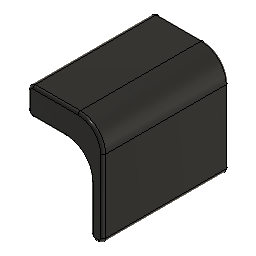
Arm Strap Support1 (Autodesk Fusion 360 design; units mm, degrees)
Autodesk Fusion 360 part; units mm, degrees
sketch "Sketch1" plane through (0, 57.15, 0) normal (0, 1, 0) x (-1, 0, 0)
  line L0 (-4.0409, -6.0198) -> (-4.0409, -7.62)
  line L1 (-4.0409, -7.62) -> (2.9359, -7.62)
  line L2 (2.9359, -7.62) -> (2.9359, -6.0198)
  line L3 (2.9359, -6.0198) -> (-4.0409, -6.0198)
  line L4 (-19.0526, 3.8099) -> (-19.0526, -5.08)
  line L5 (-21.5926, -7.62) -> (-38.1026, -7.62)
  line L6 (-50.8026, -7.62) -> (-50.8026, 6.3499)
  line L7 (-50.8026, 6.3499) -> (-21.5926, 6.3499)
  line L8 (-50.8026, -20.32) -> (-50.8026, -43.18)
  line L9 (-53.3426, -45.72) -> (-54.6126, -45.72)
  line L10 (-57.1526, -43.18) -> (-57.1526, -6.3501)
  line L11 (-44.4526, 6.3499) -> (-50.8026, 6.3499)
  arc A0 (-19.0526, 3.8099) -> (-21.5926, 6.3499) centre (-21.5926, 3.8099) ccw
  arc A1 (-21.5926, -7.62) -> (-19.0526, -5.08) centre (-21.5926, -5.08) ccw
  arc A2 (-53.3426, -45.72) -> (-50.8026, -43.18) centre (-53.3426, -43.18) ccw
  arc A3 (-57.1526, -43.18) -> (-54.6126, -45.72) centre (-54.6126, -43.18) ccw
  arc A4 (-38.1026, -7.62) -> (-50.8026, -20.32) centre (-38.1026, -20.32) ccw
  arc A5 (-44.4526, 6.3499) -> (-57.1526, -6.3501) centre (-44.4526, -6.3501) ccw
  point P0 (-19.0526, -7.62)
  point P1 (-50.8026, -45.72)
  point P2 (-57.1526, -45.72)
  dimension "d1" = 31.75
  dimension "d2" = 38.1
  dimension "d3" = 6.35
  dimension "d4" = 2.54
  dimension "d5" = 2.54
  dimension "d6" = 12.7
  constraint perpendicular L1 L4
  constraint perpendicular L4 L5
  constraint perpendicular L5 L6
  constraint perpendicular L4 L7
  constraint perpendicular L5 L8
  constraint perpendicular L8 L9
  constraint perpendicular L9 L10
  constraint perpendicular L6 L11
  constraint tangent L4 A0
  constraint tangent L7 A0
  constraint coincident P0 L4
  constraint coincident P0 L5
  constraint tangent L4 A1
  constraint tangent L5 A1
  constraint equal A0 A1
  constraint coincident P1 L8
  constraint coincident P1 L9
  constraint tangent L8 A2
  constraint tangent L9 A2
  constraint coincident P2 L9
  constraint coincident P2 L10
  constraint tangent L9 A3
  constraint tangent L10 A3
  constraint equal A2 A3
  constraint coincident L6.start L5
  constraint coincident L6.start L8
  constraint tangent L5 A4
  constraint tangent L8 A4
  constraint tangent L10 A5
  constraint tangent L11 A5
  constraint equal A4 A5
  measures "d1" distance of P0 L6.start
  measures "d2" distance of L6.start P1
  measures "d3" distance of P1 P2
  measures "d4" radius of A0
  measures "d5" radius of A2
  measures "d6" radius of A4
extrude "Extrude1" add sketch "Sketch1" against normal blind 63.5 contours L4 L5 L7 L8 L9 L10 A0 A1 A2 A3 A4 A5
hole "Hole1" at (19.0526, 0, 0) direction (1, 0, 0) diameter 3.429 depth 12.7 tip angle 180
thread "Thread1" "ANSI Unified Screw Threads 0.164(#8) 8-32 UNC 8-32 UNC 2B" major diameter 4.1656 minor diameter 3.4163 pitch 0.7937 angle 60 modelled right hand crest width 0.2341 on face at (23.2859, 0.1707, 1.706) crest through (19.251, -1.7082, 0)
hole "Hole2" at (19.0526, 25.4, 0) direction (1, 0, 0) diameter 3.429 depth 12.7 tip angle 180
thread "Thread2" "ANSI Unified Screw Threads 0.164(#8) 8-32 UNC 8-32 UNC 2B" major diameter 4.1656 minor diameter 3.4163 pitch 0.7937 angle 60 modelled right hand crest width 0.2341 on face at (23.2859, 25.5707, 1.706) crest through (19.251, 23.6918, 0)
hole "Hole3" at (19.0526, 50.8, 0) direction (1, 0, 0) diameter 3.429 depth 12.7 tip angle 180
thread "Thread3" "ANSI Unified Screw Threads 0.164(#8) 8-32 UNC 8-32 UNC 2B" major diameter 4.1656 minor diameter 3.4163 pitch 0.7937 angle 60 modelled right hand crest width 0.2341 on face at (23.2859, 50.9707, 1.706) crest through (19.251, 49.0918, 0)
fillet "Fillet1" radius 1.27 12 edges at (19.0526, -6.35, -0.6351) (19.7966, -6.35, -6.8761) (29.8476, -6.35, -7.62) (47.0829, -6.35, -11.3397) (50.8026, -6.35, -31.75) (51.5466, -6.35, -44.9761) (53.9776, -6.35, -45.72) (56.4087, -6.35, -44.9761) (57.1526, -6.35, -24.7651) (53.4329, -6.35, 2.6301) (33.0226, -6.35, 6.3499) (19.7966, -6.35, 5.6059) 1 faces at (34.7159, 57.15, 1.6932)
sketch "Sketch2" plane through (19.0526, 0, 0) normal (-1, 0, 0) x (0, -1, 0)
  line L0 (-55.88, 3.8099) -> (-55.88, -5.08)
  line L1 (-55.88, -5.08) -> (5.08, -5.08)
  line L2 (5.08, -5.08) -> (5.08, 3.8099)
  line L3 (5.08, 3.8099) -> (-55.88, 3.8099)
  spline S0 degree 3 poles (-1.0037, -1.825) (-1.2209, -1.674) (-1.4071, -1.4829) (-1.6881, -1.048) (-1.7836, -0.8108) (-1.8744, -0.3235) (-1.8728, -0.0789) (-1.7889, 0.3235) (-1.7315, 0.4832) (-1.5758, 0.7763) (-1.4795, 0.909) (-1.3657, 1.0259) knots 0 0 0 0 0.079347 0.079347 0.155456 0.155456 0.228326 0.228326 0.279114 0.279114 0.328226 0.328226 0.328226 0.328226
  arc A0 (1.3657, 1.0259) -> (-1.3657, 1.0259) centre (0, 0) ccw
  spline S1 degree 3 poles (1.3657, 1.0259) (1.5233, 0.864) (1.6469, 0.6723) (1.8197, 0.2427) (1.8634, 0.0074) (1.8602, -0.4776) (1.8092, -0.7228) (1.6412, -1.1248) (1.5443, -1.2864) (1.3049, -1.5826) (1.1624, -1.7147) (1.0037, -1.825) knots 0 0 0 0 0.06777 0.06777 0.138771 0.138771 0.213001 0.213001 0.26909 0.26909 0.326867 0.326867 0.326867 0.326867
  arc A1 (-1.0037, -1.825) -> (1.0037, -1.825) centre (0, 0) ccw
  spline S2 degree 3 poles (-26.4037, -1.825) (-26.6209, -1.674) (-26.8071, -1.4829) (-27.0881, -1.048) (-27.1836, -0.8108) (-27.2744, -0.3235) (-27.2728, -0.0789) (-27.1889, 0.3235) (-27.1315, 0.4832) (-26.9758, 0.7763) (-26.8795, 0.909) (-26.7657, 1.0259) knots 0 0 0 0 0.079347 0.079347 0.155456 0.155456 0.228326 0.228326 0.279114 0.279114 0.328226 0.328226 0.328226 0.328226
  arc A2 (-24.0343, 1.0259) -> (-26.7657, 1.0259) centre (-25.4, 0) ccw
  spline S3 degree 3 poles (-24.0343, 1.0259) (-23.8767, 0.864) (-23.7531, 0.6723) (-23.5803, 0.2427) (-23.5366, 0.0074) (-23.5398, -0.4776) (-23.5908, -0.7228) (-23.7588, -1.1248) (-23.8557, -1.2864) (-24.0951, -1.5826) (-24.2376, -1.7147) (-24.3963, -1.825) knots 0 0 0 0 0.06777 0.06777 0.138771 0.138771 0.213001 0.213001 0.26909 0.26909 0.326867 0.326867 0.326867 0.326867
  arc A3 (-26.4037, -1.825) -> (-24.3963, -1.825) centre (-25.4, 0) ccw
  spline S4 degree 3 poles (-51.8037, -1.825) (-52.0209, -1.674) (-52.2071, -1.4829) (-52.4881, -1.048) (-52.5836, -0.8108) (-52.6744, -0.3235) (-52.6728, -0.0789) (-52.5889, 0.3235) (-52.5315, 0.4832) (-52.3758, 0.7763) (-52.2795, 0.909) (-52.1657, 1.0259) knots 0 0 0 0 0.079347 0.079347 0.155456 0.155456 0.228326 0.228326 0.279114 0.279114 0.328226 0.328226 0.328226 0.328226
  arc A4 (-49.4343, 1.0259) -> (-52.1657, 1.0259) centre (-50.8, 0) ccw
  spline S5 degree 3 poles (-49.4343, 1.0259) (-49.2767, 0.864) (-49.1531, 0.6723) (-48.9803, 0.2427) (-48.9366, 0.0074) (-48.9398, -0.4776) (-48.9908, -0.7228) (-49.1588, -1.1248) (-49.2557, -1.2864) (-49.4951, -1.5826) (-49.6376, -1.7147) (-49.7963, -1.825) knots 0 0 0 0 0.06777 0.06777 0.138771 0.138771 0.213001 0.213001 0.26909 0.26909 0.326867 0.326867 0.326867 0.326867
  arc A5 (-51.8037, -1.825) -> (-49.7963, -1.825) centre (-50.8, 0) ccw
  line L4 (0, 0) -> (2.3114, 0)
  line L5 (2.3114, 0) -> (2.3114, 1.8034)
  line L6 (1.8034, 2.3114) -> (-1.8034, 2.3114)
  line L7 (-2.3114, 1.8034) -> (-2.3114, -1.8034)
  line L8 (-1.8034, -2.3114) -> (1.8034, -2.3114)
  line L9 (2.3114, -1.8034) -> (2.3114, 0)
  arc A6 (-1.8034, 2.3114) -> (-2.3114, 1.8034) centre (-1.8034, 1.8034) ccw
  arc A7 (2.3114, 1.8034) -> (1.8034, 2.3114) centre (1.8034, 1.8034) ccw
  arc A8 (1.8034, -2.3114) -> (2.3114, -1.8034) centre (1.8034, -1.8034) ccw
  arc A9 (-2.3114, -1.8034) -> (-1.8034, -2.3114) centre (-1.8034, -1.8034) ccw
  line L10 (2.2987, 0) -> (2.2987, 1.8034)
  arc A10 (2.2987, 1.8034) -> (1.8034, 2.2987) centre (1.8034, 1.8034) ccw
  line L11 (1.8034, 2.2987) -> (-1.8034, 2.2987)
  arc A11 (-1.8034, 2.2987) -> (-2.2987, 1.8034) centre (-1.8034, 1.8034) ccw
  line L12 (-2.2987, 1.8034) -> (-2.2987, -1.8034)
  arc A12 (-2.2987, -1.8034) -> (-1.8034, -2.2987) centre (-1.8034, -1.8034) ccw
  line L13 (-1.8034, -2.2987) -> (1.8034, -2.2987)
  arc A13 (1.8034, -2.2987) -> (2.2987, -1.8034) centre (1.8034, -1.8034) ccw
  line L14 (2.2987, -1.8034) -> (2.2987, 0)
  line L15 (-2.0447, 1.8034) -> (-2.0447, -1.8034)
  arc A14 (-2.0447, -1.8034) -> (-1.8034, -2.0447) centre (-1.8034, -1.8034) ccw
  line L16 (-1.8034, -2.0447) -> (1.8034, -2.0447)
  arc A15 (1.8034, -2.0447) -> (2.0447, -1.8034) centre (1.8034, -1.8034) ccw
  line L17 (2.0447, -1.8034) -> (2.0447, 0)
  line L18 (2.0447, 0) -> (2.0447, 1.8034)
  arc A16 (2.0447, 1.8034) -> (1.8034, 2.0447) centre (1.8034, 1.8034) ccw
  line L19 (1.8034, 2.0447) -> (-1.8034, 2.0447)
  arc A17 (-1.8034, 2.0447) -> (-2.0447, 1.8034) centre (-1.8034, 1.8034) ccw
  line L20 (-23.5966, 2.0447) -> (-27.2034, 2.0447)
  arc A18 (-27.2034, 2.0447) -> (-27.4447, 1.8034) centre (-27.2034, 1.8034) ccw
  line L21 (-27.4447, 1.8034) -> (-27.4447, -1.8034)
  arc A19 (-27.4447, -1.8034) -> (-27.2034, -2.0447) centre (-27.2034, -1.8034) ccw
  line L22 (-27.2034, -2.0447) -> (-23.5966, -2.0447)
  line L23 (-23.3553, -1.8034) -> (-23.3553, 0)
  arc A20 (-23.5966, -2.0447) -> (-23.3553, -1.8034) centre (-23.5966, -1.8034) ccw
  line L24 (-23.3553, 0) -> (-23.3553, 1.8034)
  arc A21 (-23.3553, 1.8034) -> (-23.5966, 2.0447) centre (-23.5966, 1.8034) ccw
  line L25 (-23.5966, 2.2987) -> (-27.2034, 2.2987)
  arc A22 (-23.1013, 1.8034) -> (-23.5966, 2.2987) centre (-23.5966, 1.8034) ccw
  line L26 (-23.1013, 0) -> (-23.1013, 1.8034)
  line L27 (-23.1013, -1.8034) -> (-23.1013, 0)
  arc A23 (-23.5966, -2.2987) -> (-23.1013, -1.8034) centre (-23.5966, -1.8034) ccw
  line L28 (-27.2034, -2.2987) -> (-23.5966, -2.2987)
  arc A24 (-27.6987, -1.8034) -> (-27.2034, -2.2987) centre (-27.2034, -1.8034) ccw
  line L29 (-27.6987, 1.8034) -> (-27.6987, -1.8034)
  arc A25 (-27.2034, 2.2987) -> (-27.6987, 1.8034) centre (-27.2034, 1.8034) ccw
  line L30 (-48.9966, 2.0447) -> (-52.6034, 2.0447)
  arc A26 (-52.6034, 2.0447) -> (-52.8447, 1.8034) centre (-52.6034, 1.8034) ccw
  line L31 (-52.8447, 1.8034) -> (-52.8447, -1.8034)
  arc A27 (-52.8447, -1.8034) -> (-52.6034, -2.0447) centre (-52.6034, -1.8034) ccw
  line L32 (-52.6034, -2.0447) -> (-48.9966, -2.0447)
  line L33 (-48.7553, -1.8034) -> (-48.7553, 0)
  arc A28 (-48.9966, -2.0447) -> (-48.7553, -1.8034) centre (-48.9966, -1.8034) ccw
  line L34 (-48.7553, 0) -> (-48.7553, 1.8034)
  arc A29 (-48.7553, 1.8034) -> (-48.9966, 2.0447) centre (-48.9966, 1.8034) ccw
  line L35 (-48.9966, 2.2987) -> (-52.6034, 2.2987)
  arc A30 (-48.5013, 1.8034) -> (-48.9966, 2.2987) centre (-48.9966, 1.8034) ccw
  line L36 (-48.5013, 0) -> (-48.5013, 1.8034)
  line L37 (-48.5013, -1.8034) -> (-48.5013, 0)
  arc A31 (-48.9966, -2.2987) -> (-48.5013, -1.8034) centre (-48.9966, -1.8034) ccw
  line L38 (-52.6034, -2.2987) -> (-48.9966, -2.2987)
  arc A32 (-53.0987, -1.8034) -> (-52.6034, -2.2987) centre (-52.6034, -1.8034) ccw
  line L39 (-53.0987, 1.8034) -> (-53.0987, -1.8034)
  arc A33 (-52.6034, 2.2987) -> (-53.0987, 1.8034) centre (-52.6034, 1.8034) ccw
  point P0 (2.3114, 2.3114)
  point P1 (-2.3114, 2.3114)
  point P2 (-2.3114, -2.3114)
  point P3 (2.3114, -2.3114)
  dimension "d30" = 2.3114
  dimension "d31" = 2.3114
  dimension "d32" = 4.6228
  dimension "d33" = 4.6228
  dimension "d34" = 4.6228
  dimension "d35" = 0.508
  dimension "d36" = -0.0127
  dimension "d37" = -0.254
  dimension "d42" = -50.8
  dimension "d43" = 0
  constraint horizontal L4
  constraint coincident A0.centre A1.centre
  constraint perpendicular L4 L5
  constraint perpendicular L5 L6
  constraint perpendicular L6 L7
  constraint perpendicular L7 L8
  constraint coincident P1 L6
  constraint coincident P1 L7
  constraint tangent L6 A6
  constraint tangent L7 A6
  constraint coincident P0 L6
  constraint coincident P0 L5
  constraint tangent L6 A7
  constraint tangent L5 A7
  constraint equal A6 A7
  constraint coincident P3 L8
  constraint coincident P3 L9
  constraint tangent L8 A8
  constraint tangent L9 A8
  constraint equal A6 A8
  constraint coincident P2 L7
  constraint coincident P2 L8
  constraint tangent L7 A9
  constraint tangent L8 A9
  constraint equal A6 A9
  measures "d30" distance of A0.centre L4.end
  measures "d31" distance of L4.end P0
  measures "d32" distance of P0 P1
  measures "d33" distance of P1 P2
  measures "d34" distance of P2 P3
  measures "d35" radius of A6
equation "d32 = ( 0.091 * 2 ) * 1 in"
equation "d33 = ( 0.091 * 2 ) * 1 in"
equation "d34 = ( 0.091 * 2 ) * 1 in"
named bodies: "ArmSupport1"
